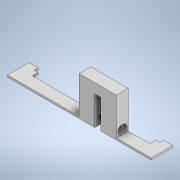
# Autodesk Inventor part: screw_supp
Saved by Autodesk Inventor 2020 (Build 240168000, 168)
## iProperties
Created: 2019-12-09
Part Number: screw_supp
Material: Generic
Document SubType Name: Modeling
Designer: sl65b
Density: 1 g/cm^3
Appearance: Default
Author: sl65b
Autodesk Inventor part; units mm, degrees
ref_plane "YZ Plane" through (0, 0, 0) normal (1, 0, 0) x (0, 1, 0)
ref_plane "XZ Plane" through (0, 0, 0) normal (0, 1, 0) x (-1, 0, 0)
ref_plane "XY Plane" through (0, 0, 0) normal (0, 0, 1) x (1, 0, 0)
sketch "Sketch1" plane through (0, 0, 0) normal (0, 1, 0) x (-1, 0, 0)
  line L0 (-62.1475, 5) -> (-62.1475, 11)
  line L1 (-62.1475, 11) -> (-2.0643, 11)
  line L2 (-2.0643, 5) -> (-2.0643, 11)
  line L3 (-2.0643, 11) -> (-62.1475, 11)
  line L4 (-2.0643, 5) -> (-62.1475, 5)
  line L5 (-4.3424, 5) -> (-59.9525, 5)
  line L6 (-62.1475, 11) -> (-2.0643, 11)
  line L7 (-43.2275, 5) -> (-43.2275, 11)
  line L8 (-40.0775, 5) -> (-40.0775, 11)
  line L9 (-62.2307, 5) -> (-2.0643, 5)
  line L10 (-32.0775, 5) -> (-32.0775, 11)
  line L11 (-51.2275, 5) -> (-51.2275, 11)
  point P0 (0, 0)
  dimension "d0" = 18.92
  dimension "d1" = 3.15
  dimension "d2" = 8
  dimension "d3" = 8
  constraints: 24 end point, 8 point on line, 4 perpendicular, 2 parallel, 1 collinear, 1 vertical
  measures "d0" distance between parallel lines of L0 L7
  measures "d1" distance between parallel lines of L8 L7
  measures "d2" distance between parallel lines of L8 L10
  measures "d3" distance between parallel lines of L11 L7
extrude "Extrusion1" add sketch "Sketch1" along normal blind 20 contours L1 L7 L4 L11 | L1 L10 L4 L8
sketch "Sketch2" plane through (0, 0, 0) normal (0, 1, 0) x (-1, 0, 0)
  line L0 (4.7021, 0) -> (4.7021, 5)
  line L1 (4.7021, 0) -> (4.7021, 11)
  line L2 (-32.0775, 11) -> (4.7021, 11)
  line L3 (4.7021, 11) -> (-32.0775, 11)
  line L4 (-32.0775, 11) -> (-32.0775, 5)
  line L5 (-4.3424, 5) -> (-2.0643, 5)
  line L6 (-32.0775, 5) -> (-2.0643, 5)
  line L7 (-2.0643, 5) -> (-2.0643, 2)
  line L8 (0, 2) -> (-2.0643, 2)
  line L9 (-2.0643, 2) -> (0, 2)
  line L10 (0, 2) -> (0, 0)
  line L11 (4.7021, 0) -> (0, 0)
  line L12 (0, 0) -> (4.7021, 0)
  line L13 (-51.2275, 5) -> (-51.2275, 11)
  line L14 (-51.2275, 5) -> (-51.2275, 11)
  line L15 (-69.0002, 11) -> (-51.2275, 11)
  line L16 (-51.2275, 11) -> (-69.0002, 11)
  line L17 (-69.0002, 0) -> (-69.0002, 5)
  line L18 (-69.0002, 11) -> (-69.0002, 0)
  line L19 (4.7021, 0) -> (0, 0)
  line L20 (-69.0002, 0) -> (-64.295, 0)
  line L21 (-64.295, 0) -> (-64.295, 1.7012)
  line L22 (0, 2) -> (-2.0643, 2)
  line L23 (-2.0643, 2) -> (-2.0643, 5)
  line L24 (-62.2307, 2) -> (-62.2307, 5)
  line L25 (-62.2307, 5) -> (-51.2275, 5)
  line L26 (-64.295, 2) -> (-62.2307, 2)
  line L27 (-64.295, 2) -> (-64.295, 1.7012)
  point P0 (-68.997, 0)
  constraints: 54 end point, 8 perpendicular, 3 collinear, 2 horizontal, 2 parallel, 1 vertical, 3 other
extrude "Extrusion2" add sketch "Sketch2" along normal blind 1
sketch "Sketch3" plane through (40.0775, 0, 11) normal (1, 0, 0) x (0, 0, -1)
  line L0 (6, 1) -> (6, 20) projected
  line L1 (6, 20) -> (6, 15)
  line L2 (6, 15) -> (0, 15)
  line L3 (0, 1) -> (0, 20) projected
  line L4 (0, 20) -> (6, 20)
  point P0 (11, 0)
  dimension "d8" = 5
  constraints: 6 end point, 2 point on line, 1 parallel, 1 perpendicular
  measures "d8" distance of L0.end L1.end
extrude "Extrusion3" add sketch "Sketch3" along normal blind 5.5
sketch "Sketch4" plane through (51.2275, 20, 11) normal (1, 0, 0) x (0, 0, -1)
  line L0 (6, -19) -> (6, 0) projected
  line L1 (0, -19) -> (0, 0) projected
  circle A0 centre (3, -16.8) radius 0.9682
  line L2 (0, -19) -> (11, -19) projected
  point P0 (11, -20)
  dimension "d11" = 6
  dimension "d12" = 3
  dimension "d13" = 2.2
  constraints: 1 centre point
  measures "d11" distance between parallel lines of L0 L1
  measures "d12" distance from line of L0 A0.centre
  measures "d13" distance from line of L2 A0.centre
hole "Hole1" at (51.2275, 3.2, 8) direction (-1, 0, 0) diameter 2.4 depth 24 tip angle 118 counterbore diameter 4.6 counterbore depth 1.5
body "Solid1"
